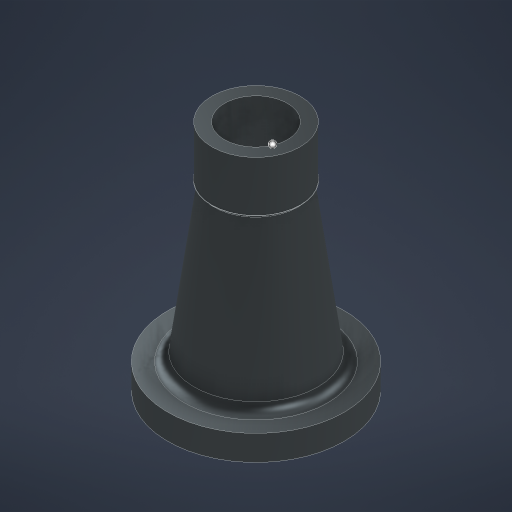
# Autodesk Inventor part: body
Saved by Autodesk Inventor 2023 (Build 270158000, 158)
## iProperties
Created: 2023-03-09
Part Number: body
Material: Iron, Cast
Document SubType Name: Modeling
Designer: kamra
Density: 7.15 g/cm^3
Appearance: Iron Gray
Author: kamra
Autodesk Inventor part; units mm, degrees
ref_plane "YZ Plane" through (0, 0, 0) normal (1, 0, 0) x (0, 1, 0)
ref_plane "XZ Plane" through (0, 0, 0) normal (0, 1, 0) x (-1, 0, 0)
ref_plane "XY Plane" through (0, 0, 0) normal (0, 0, 1) x (1, 0, 0)
sketch "FV.sec" plane through (0, 0, 0) normal (0, 0, 1) x (1, 0, 0)
  line L0 (25, 185) -> (35, 185)
  line L1 (35, 185) -> (35, 145)
  line L2 (25, 185) -> (25, 129.6172)
  line L3 (50, 20) -> (70, 20)
  line L4 (70, 20) -> (70, 0)
  line L5 (0, 0) -> (0, 185)
  line L6 (35, 145) -> (35.2904, 145)
  line L7 (33.3087, 142.7305) -> (50, 20)
  line L8 (70, 0) -> (50, 0)
  line L9 (50, 0) -> (50, 3)
  line L10 (50, 3) -> (42.2199, 3)
  line L11 (42.2199, 3) -> (25, 129.6172)
  arc A0 (35.2904, 145) -> (33.3087, 142.7305) centre (35.2904, 143) ccw
  point P0 (33, 145)
  dimension "d9" = 40
  dimension "d11" = 185
  dimension "d12" = 20
  dimension "d16" = 3
  dimension "d17" = 10
  dimension "d18" = 66
  dimension "d21" = 100
  dimension "d22" = 10
  dimension "d23" = 100
  dimension "d24" = 20
  dimension "d28" = 2
  constraints: 24 end point, 4 horizontal, 3 perpendicular, 3 point on line, 2 parallel, 2 point on circle, 2 tangent, 2 vertical, 1 centre point, 1 horizontal alignment
  measures "d9" distance of L0.end L1.end
  measures "d11" distance from line of L4.end L0
  measures "d12" distance of L3.end L4.end
  measures "d16" distance of L8.end L9.end
  measures "d17" distance between parallel lines of L7 L11
  measures "d18" diameter of point (33, 145) L5
  measures "d21" diameter of L9 L5
  measures "d22" distance of L0.start L0.end
  measures "d23" diameter of L3.start L5
  measures "d24" distance of L4.end L8.end
  measures "d28" radius of A0
revolve "Revolution1" add sketch "FV.sec" angle 360 about axis through (0, 0, 0) along (0, 1, 0)
fillet "Fillet1" radius 8 1 edges at (-50, 20, 0)
